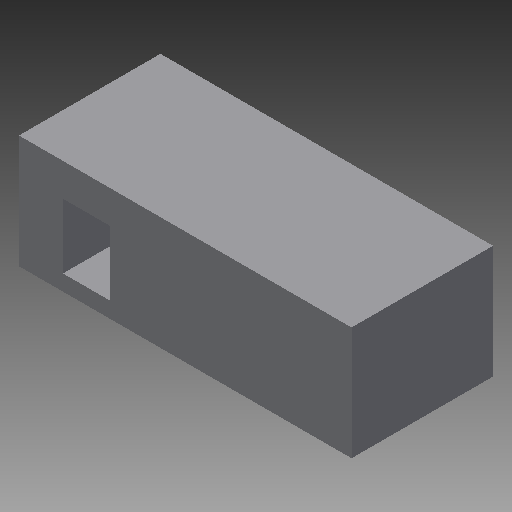
# Autodesk Inventor part: frame2
Saved by Autodesk Inventor 2017 (Build 210142000, 142)
## iProperties
Created: 2016-10-09
Part Number: frame2
Material: Generic
Document SubType Name: Modeling
Designer: Paulo Loma
Density: 1 g/cm^3
Appearance: Default
Author: Paulo Loma
Autodesk Inventor part; units mm, degrees
ref_plane "YZ Plane" through (0, 0, 0) normal (1, 0, 0) x (0, 1, 0)
ref_plane "XZ Plane" through (0, 0, 0) normal (0, 1, 0) x (-1, 0, 0)
sketch "Sketch1" plane through (0, 0, 0) normal (0, 0, 1) x (1, 0, 0)
  line L0 (0, 5.1) -> (0, 10.2)
  line L1 (38.3, 5.1) -> (38.3, 10.2)
  line L2 (0, 0) -> (0, 5.1)
  line L3 (38.3, 0) -> (38.3, 5.1)
  line L4 (40.3, -1) -> (40.3, 11.2)
  line L5 (40.3, -1) -> (40.3, -2)
  line L6 (40.3, -2) -> (-1, -2)
  line L7 (-1, -2) -> (-2, -2)
  line L8 (-2, -2) -> (-2, 11.2)
  line L9 (38.3, 5.1) -> (38.3, 10.4)
  line L10 (38.3, 10.4) -> (0, 10.4)
  line L11 (0, 10.4) -> (0, 5.1)
  line L12 (0, 12.4) -> (-2, 12.4)
  line L13 (-2, 12.4) -> (-2, 11.2)
  line L14 (0, 12.4) -> (40.3, 12.4)
  line L15 (40.3, 12.4) -> (40.3, 11.2)
  line L16 (38.3, 0) -> (38.3, -2)
  line L17 (0, 0) -> (0, -2)
  dimension "d108" = 5.3
  constraints: 36 end point, 8 perpendicular, 5 point on line, 1 collinear, 1 horizontal, 1 vertical
  measures "d108" distance of L1.start L9.end
extrude "Extrusion1" add sketch "Sketch1" against normal blind 12 contours L2 L17 L6 L7 L8 L13 L12 L14 L15 L4 L5 L16 L3 L1 L9 L10 L11 L0
sketch "Sketch2" plane through (0, 0, 0) normal (0, 0, 1) x (1, 0, 0)
  line L0 (3.5908, 8.23) -> (9.5908, 8.23)
  line L1 (9.5908, 8.23) -> (9.5908, 0)
  line L2 (3.5908, 0) -> (9.5908, 0)
  line L3 (3.5908, 8.23) -> (3.5908, 0)
  line L4 (40.3, 12.4) -> (-2, 12.4)
  line L5 (-2, 12.4) -> (-2, -2)
  line L6 (-2, -2) -> (15, -2)
  line L7 (15, -2) -> (40.3, -2)
  line L8 (38.3, -2) -> (40.3, -2) projected
  line L9 (40.3, -2) -> (40.3, 12.4)
  line L10 (40.3, -2) -> (40.3, 12.4) projected
  point P0 (39.3, 11.2)
  point P1 (15, 12.4)
  dimension "d4" = 6
  constraints: 18 end point, 2 collinear, 1 point on line
  measures "d4" distance of L0.start L0.end
ref_plane "Work Plane10" through (0, 5.1, -62.2) normal (0, 0, -1) x (0, 1, 0)
sketch "Sketch20" plane through (0, -2, -12) normal (1, 0, 0) x (0, 0, -1)
  line L0 (0, 14.4) -> (0, 0) projected
  line L1 (0, 2) -> (0, 0)
  line L2 (0, 0) -> (-12, 0)
  line L3 (-12, 0) -> (0, 0) projected
  line L4 (-12, 0) -> (-12, 2)
  line L5 (-12, 2) -> (0, 2)
  constraints: 8 end point, 2 collinear, 2 perpendicular, 1 point on line
extrude "Extrusion25" add sketch "Sketch20" along normal blind 1
sketch "Sketch21" plane through (38.3, -2, 0) normal (-1, 0, 0) x (0, 0, 1)
  line L0 (0, 2) -> (0, 0)
  line L1 (-12, 0) -> (-12, 2)
  line L2 (-12, 14.4) -> (-12, 0) projected
  line L3 (0, 2) -> (0, 0)
  line L4 (-12, 2) -> (0, 2)
  line L5 (0, 2) -> (2.5, 2) projected
  line L6 (0, 2) -> (0, 0)
  line L7 (0, 0) -> (-12, 0)
  line L8 (0, 0) -> (-12, 0) projected
  constraints: 12 end point, 2 collinear, 1 parallel, 1 perpendicular, 1 point on line, 1 vertical
extrude "Extrusion26" add sketch "Sketch21" along normal blind 1
extrude "Extrusion27" add sketch "Sketch2" along normal blind 6
body "Solid1"
